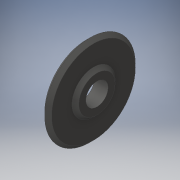
# Autodesk Inventor part: idler_spacer
Saved by Autodesk Inventor 2016 (Build 200138000, 138)
## iProperties
Created: 2016-06-04
Part Number: idler_spacer
Material: Generic
Document SubType Name: Modeling
Designer: brent
Density: 1 g/cm^3
Appearance: Generic
Author: brent
Autodesk Inventor part; units mm, degrees
ref_plane "YZ Plane" through (0, 0, 0) normal (1, 0, 0) x (0, 1, 0)
ref_plane "XZ Plane" through (0, 0, 0) normal (0, 1, 0) x (-1, 0, 0)
ref_plane "XY Plane" through (0, 0, 0) normal (0, 0, 1) x (1, 0, 0)
sketch "Sketch1" plane through (0, 0, 0) normal (0, 1, 0) x (-1, 0, 0)
  line L0 (0, 0) -> (1, 0)
  line L1 (1, 0) -> (1, -6.5)
  line L2 (1, -6.5) -> (0, -6.5)
  line L3 (0, -6.5) -> (0, 0)
  line L4 (1, 0) -> (0, 0)
  line L5 (0, 0) -> (0, -1.6)
  line L6 (0, -1.6) -> (1, -1.6)
  line L7 (1, -1.6) -> (1, 0)
  line L8 (1, -1.6) -> (1.5, -1.6)
  line L9 (1.5, -1.6) -> (1.5, -2.6)
  line L10 (1.5, -2.6) -> (1, -2.6)
  line L11 (1, -2.6) -> (1, -1.6)
  line L12 (0, -1.6) -> (-0.5, -1.6)
  line L13 (-0.5, -1.6) -> (-0.5, -2.6)
  line L14 (-0.5, -2.6) -> (0, -2.6)
  line L15 (0, -2.6) -> (0, -1.6)
  dimension "d0" = 1
  dimension "d1" = 6.5
  dimension "d2" = 1.6
  dimension "d3" = 0.5
  dimension "d4" = 1
  dimension "d5" = 0.5
  dimension "d6" = 1
  constraints: 32 end point, 8 parallel, 4 horizontal, 4 perpendicular, 1 point on line
  measures "d0" distance of L1.end L2.end
  measures "d1" distance of L0.end L1.end
  measures "d2" distance of L5.end L4.end
  measures "d3" distance of L9.end L10.end
  measures "d4" distance of L8.end L9.end
  measures "d5" distance of L14.end L13.end
  measures "d6" distance of L13.end L12.end
revolve "Revolution1" add sketch "Sketch1" angle 360 about axis through (0, 0, 0) along (-1, 0, 0) contours L6 L1 L2 L3 | L3 L14 L13 L12 | L8 L9 L10 L1
chamfer "Chamfer1" distance 0.5 angle 45 4 edges at (-1, 0, 2.6) (0, 0, 2.6) (0, 0, 6.5) (-1, 0, 6.5)
body "Solid1"
